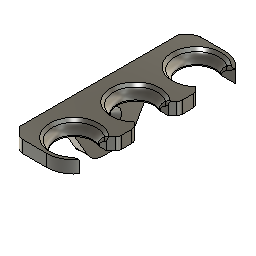
SKADIS_SNS_WeraMicro (Autodesk Fusion 360 design; units mm, degrees)
Autodesk Fusion 360 part; units mm, degrees
sketch "SlotLayout" plane through (0, 0, 0) normal (1, 0, 0) x (0, 1, 0)
  line L0 (-22.4, 25) -> (-22.4, 15)
  line L1 (82.4, 5) -> (82.4, -5)
  line L2 (-37.6, -5) -> (-37.6, 5)
  line L3 (-80, 5) -> (-80, -5) construction
  line L4 (-97.6, 15) -> (-97.6, 25)
  line L5 (2.4, -5) -> (2.4, 5)
  arc A0 (-77.6, 5) -> (-82.4, 5) centre (-80, 5) ccw
  arc A1 (22.4, 25) -> (17.6, 25) centre (20, 25) ccw
  arc A2 (-97.6, 25) -> (-102.4, 25) centre (-100, 25) ccw
  arc A3 (97.6, 15) -> (102.4, 15) centre (100, 15) ccw
  line L6 (-60, 25) -> (-60, 15) construction
  line L7 (-77.6, -5) -> (-77.6, 5)
  arc A4 (77.6, -5) -> (82.4, -5) centre (80, -5) ccw
  line L8 (-40, 5) -> (-40, -5) construction
  line L9 (-57.6, 15) -> (-57.6, 25)
  line L10 (-62.4, 25) -> (-62.4, 15)
  line L11 (-102.4, 25) -> (-102.4, 15)
  line L12 (97.6, 15) -> (97.6, 25)
  arc A5 (-102.4, 15) -> (-97.6, 15) centre (-100, 15) ccw
  line L13 (20, 25) -> (20, 15) construction
  line L14 (22.4, 25) -> (22.4, 15)
  line L15 (-80, 0) -> (0, 0) construction
  line L16 (62.4, 25) -> (62.4, 15)
  line L17 (42.4, 5) -> (42.4, -5)
  arc A6 (2.5, 5) -> (-2.5, 5) centre (0, 5) ccw
  arc A7 (2.4, 5) -> (-2.4, 5) centre (0, 5) ccw
  line L18 (80, 5) -> (80, -5) construction
  arc A8 (82.4, 5) -> (77.6, 5) centre (80, 5) ccw
  arc A9 (-2.5, -5) -> (2.5, -5) centre (0, -5) ccw
  arc A10 (57.6, 15) -> (62.4, 15) centre (60, 15) ccw
  arc A11 (62.4, 25) -> (57.6, 25) centre (60, 25) ccw
  line L19 (17.6, 15) -> (17.6, 25)
  line L20 (-20, 25) -> (-20, 15) construction
  line L21 (-42.4, 5) -> (-42.4, -5)
  line L22 (60, 25) -> (60, 15) construction
  arc A12 (42.4, 5) -> (37.6, 5) centre (40, 5) ccw
  line L23 (-100, 25) -> (-100, 15) construction
  line L24 (100, 25) -> (100, 15) construction
  arc A13 (-57.6, 25) -> (-62.4, 25) centre (-60, 25) ccw
  arc A14 (37.6, -5) -> (42.4, -5) centre (40, -5) ccw
  line L25 (40, 5) -> (40, -5) construction
  line L26 (-17.6, 15) -> (-17.6, 25)
  arc A15 (-17.6, 25) -> (-22.4, 25) centre (-20, 25) ccw
  line L27 (-82.4, 5) -> (-82.4, -5)
  line L28 (-2.5, 5) -> (-2.5, -5)
  line L29 (-2.4, 5) -> (-2.4, -5)
  line L30 (102.4, 25) -> (102.4, 15)
  arc A16 (17.6, 15) -> (22.4, 15) centre (20, 15) ccw
  arc A17 (-22.4, 15) -> (-17.6, 15) centre (-20, 15) ccw
  line L31 (37.6, -5) -> (37.6, 5)
  line L32 (0, 5) -> (0, -5) construction
  arc A18 (-62.4, 15) -> (-57.6, 15) centre (-60, 15) ccw
  arc A19 (-42.4, -5) -> (-37.6, -5) centre (-40, -5) ccw
  arc A20 (-2.4, -5) -> (2.4, -5) centre (0, -5) ccw
  arc A21 (102.4, 25) -> (97.6, 25) centre (100, 25) ccw
  arc A22 (-82.4, -5) -> (-77.6, -5) centre (-80, -5) ccw
  arc A23 (-37.6, 5) -> (-42.4, 5) centre (-40, 5) ccw
  line L33 (77.6, -5) -> (77.6, 5)
  line L34 (57.6, 15) -> (57.6, 25)
  line L35 (2.5, -5) -> (2.5, 5)
  point P0 (-20, 20)
  point P1 (-40, 0)
  dimension "d9" = -40
  dimension "d10" = 0
  dimension "d255" = 0.1
  dimension "d22" = 10
  dimension "d23" = 2.4
  dimension "d4" = 40
  dimension "d25" = 40
  dimension "d26" = 20
  dimension "d27" = 20
  constraint tangent L27 A22
  constraint tangent L7 A22
  constraint parallel L7 L27
  constraint tangent A0 L7
  constraint tangent A0 L27
  constraint vertical L3
  constraint tangent L21 A19
  constraint tangent L2 A19
  constraint parallel L2 L21
  constraint tangent L2 A23
  constraint tangent L21 A23
  constraint vertical L8
  constraint tangent L29 A20
  constraint tangent L5 A20
  constraint parallel L5 L29
  constraint tangent L5 A7
  constraint tangent A7 L29
  constraint parallel L2 L32
  constraint midpoint L15.start L3
  constraint midpoint L15.end L32
  constraint horizontal L15
  constraint equal L8 L32
  constraint equal L3 L8
  constraint midpoint P1 L8
  constraint coincident P1 L15
  constraint equal A7 A23
  constraint equal A0 A23
  constraint coincident L15.end origin
  constraint symmetric A0.end L1.start L32
  constraint symmetric L1.end L27.end L32
  constraint symmetric L7.start A4.start L32
  constraint symmetric A8.end A0.start L32
  constraint symmetric A4 L32 A22
  constraint symmetric A0 A8 L32
  constraint symmetric L17.start L21.start L32
  constraint symmetric L17.end L21.end L32
  constraint symmetric A14.start L2.start L32
  constraint symmetric A12.end L2.end L32
  constraint symmetric A14 L32 A19
  constraint symmetric A12 L32 A23
  constraint tangent L0 A17
  constraint tangent L26 A17
  constraint parallel L0 L26
  constraint tangent L26 A15
  constraint tangent L0 A15
  constraint vertical L20
  constraint equal L20 L32
  constraint equal A7 A15
  constraint midpoint P0 L20
  constraint symmetric L0.end L14.end L32
  constraint symmetric L26.end A1.end L32
  constraint symmetric L0.start A1.start L32
  constraint symmetric L26.start L19.start L32
  constraint symmetric A1 A15 L32
  constraint symmetric A16 A17 L32
  constraint symmetric A11.end L9.end L32
  constraint symmetric L16.start L10.start L32
  constraint symmetric A11 A13 L32
  constraint symmetric L16.end L10.end L32
  constraint symmetric A10.start L9.start L32
  constraint symmetric A10 L32 A18
  constraint symmetric L12.end L4.end L32
  constraint symmetric L30.start A2.end L32
  constraint symmetric A2 L32 A21
  constraint symmetric A3.end L11.end L32
  constraint symmetric A3.start L4.start L32
  constraint symmetric A3 A5 L32
  measures "d22" distance of A6.centre A9.centre
  measures "d23" radius of A7
  measures "d4" distance of L8 L32
  measures "d25" distance of L3 L8
  measures "d26" horizontal distance of L20.end A6.centre
  measures "d27" vertical distance of P0 L15.end
sketch "VerticalPrintKey" plane through (0, 0, 0) normal (1, 0, 0) x (0, 1, 0)
  line L0 (-2.6, 6.7) -> (2.6, 6.7)
  line L1 (2.6, 6.7) -> (2.6, -6.7)
  line L2 (2.6, -6.7) -> (-2.6, -6.7)
  line L3 (-2.6, -6.7) -> (-2.6, 6.7)
  line L4 (0, 6.7) -> (0, -6.7) construction
  circle A0 centre (0, 0) radius 1.6
  line L5 (2.6, 0) -> (20.8722, 0) construction
  line L6 (20.8722, 0) -> (11.7361, 9.1361) construction
  line L7 (11.7361, 9.1361) -> (11.7361, -9.1361) construction
  line L8 (11.7361, -9.1361) -> (20.8722, 0) construction
  dimension "d18" = 13.4
  dimension "d19" = 5.2
  dimension "d20" = 3.2
  constraint horizontal L0
  constraint vertical L1
  constraint horizontal L2
  constraint vertical L3
  constraint midpoint L0 L4.start
  constraint midpoint L2 L4.end
  constraint midpoint L4 A0.centre
  constraint coincident A0.centre origin
  constraint midpoint L1 L5.start
  constraint perpendicular L1 L5
  constraint perpendicular L5 L7
  constraint perpendicular L6 L8
  constraint midpoint L5 L7
  measures "d18" distance of L4.start L4.end
  measures "d19" distance of L1 L3
  measures "d20" diameter of A0
sketch "HorizontalPrintKey" plane through (0, 0, 0) normal (1, 0, 0) x (0, 1, 0)
  circle A0 centre (0, 0) radius 1.6
  line L0 (2.6, -6.7) -> (-2.6, -6.7)
  line L1 (-2.6, -6.7) -> (-2.6, 6.7)
  line L2 (-2.6, 6.7) -> (2.6, 6.7)
  line L3 (2.6, 6.7) -> (2.6, -6.7)
  line L4 (0, 6.7) -> (0, -6.7) construction
  line L5 (0, 6.7) -> (0, 23.5939) construction
  line L6 (0, 23.5939) -> (-8.4469, 15.1469) construction
  line L7 (-8.4469, 15.1469) -> (8.4469, 15.1469) construction
  line L8 (8.4469, 15.1469) -> (0, 23.5939) construction
  line L9 (17.4, -6.7) -> (17.4, 6.7)
  line L10 (17.4, 6.7) -> (22.6, 6.7)
  line L11 (22.6, -6.7) -> (17.4, -6.7)
  line L12 (22.6, 6.7) -> (22.6, -6.7)
  circle A1 centre (20, 0) radius 1.6
  line L13 (37.4, -6.7) -> (37.4, 6.7)
  line L14 (37.4, 6.7) -> (42.6, 6.7)
  line L15 (42.6, -6.7) -> (37.4, -6.7)
  line L16 (42.6, 6.7) -> (42.6, -6.7)
  circle A2 centre (40, 0) radius 1.6
  line L17 (-37.4, 6.7) -> (-42.6, 6.7)
  line L18 (-22.6, -6.7) -> (-17.4, -6.7)
  line L19 (-42.6, -6.7) -> (-37.4, -6.7)
  line L20 (-37.4, -6.7) -> (-37.4, 6.7)
  circle A3 centre (-40, 0) radius 1.6
  circle A4 centre (-20, 0) radius 1.6
  line L21 (-42.6, 6.7) -> (-42.6, -6.7)
  line L22 (-22.6, 6.7) -> (-22.6, -6.7)
  line L23 (-17.4, -6.7) -> (-17.4, 6.7)
  line L24 (-17.4, 6.7) -> (-22.6, 6.7)
  dimension "d21" = 13.4
  dimension "d24" = 5.2
  dimension "d28" = 3.2
  dimension "d32" = 20
  dimension "d33" = 0
  constraint horizontal L2
  constraint vertical L3
  constraint horizontal L0
  constraint vertical L1
  constraint midpoint L4.start L2
  constraint midpoint L4.end L0
  constraint midpoint A0.centre L4
  constraint coincident A0.centre origin
  constraint perpendicular L2 L5
  constraint perpendicular L5 L7
  constraint midpoint L5 L7
  constraint perpendicular L6 L8
  constraint symmetric L5 L9.start L18.end
  constraint symmetric L5 L9.end L23.end
  constraint symmetric L5 L10.end L22.start
  constraint symmetric L5 L11.start L18.start
  constraint symmetric L5 A1 A4
  constraint symmetric L5 L13.start L19.end
  constraint symmetric L5 L13.end L17.start
  constraint symmetric L5 L14.end L17.end
  constraint symmetric L5 L15.start L19.start
  constraint symmetric L5 A2 A3
  measures "d21" distance of L4.end L4.start
  measures "d24" distance of L1 L3
  measures "d28" diameter of A0
sketch "MainProfile " plane through (0, 0, 0) normal (0, 0, 1) x (1, 0, 0) in component "SNS_WeraMicro_x3"
  circle A0 centre (12, 20) radius 9 construction
  arc A1 (12, -29) -> (19.1239, -25.5) centre (12, -20) ccw
  line L0 (14.3979, -14.5) -> (19.1239, -14.5)
  line L1 (0, 29) -> (12, 29)
  line L2 (0, 0) -> (0, -29)
  line L3 (12, -20) -> (12, 20) construction
  circle A2 centre (12, -20) radius 9 construction
  line L4 (4, 29) -> (4, -29)
  line L5 (14.3979, 14.5) -> (19.1239, 14.5)
  line L6 (14.3979, 5.5) -> (19.1239, 5.5)
  arc A3 (19.1239, 25.5) -> (12, 29) centre (12, 20) ccw
  line L7 (14.3979, -25.5) -> (19.1239, -25.5)
  circle A4 centre (12, -20) radius 6
  line L8 (0, 0) -> (0, 29)
  line L9 (14.3979, -5.5) -> (19.1239, -5.5)
  line L10 (19.1239, -25.5) -> (19.1239, 25.5)
  line L11 (19.1239, 25.5) -> (14.3979, 25.5)
  line L12 (12, 0) -> (0, 0) construction
  circle A5 centre (12, 0) radius 9 construction
  line L13 (0, -29) -> (12, -29)
  circle A6 centre (12, 20) radius 6
  circle A7 centre (12, 0) radius 6
  dimension "d34" = 12
  dimension "d5" = 40
  dimension "d6" = 18
  dimension "d37" = 12
  dimension "d38" = 5.5
  dimension "d13" = 4
  constraint vertical L3
  constraint coincident L12.start L3
  constraint coincident L2.start L8.start
  constraint midpoint L12.start L3
  constraint horizontal L12
  constraint coincident A1.centre L3.start
  constraint coincident L12.start A5.centre
  constraint coincident A0.centre L3.end
  constraint equal A4 A7
  constraint equal A6 A7
  constraint concentric A2 A4
  constraint concentric A5 A7
  constraint concentric A0 A6
  constraint equal A0 A5
  constraint equal A2 A5
  constraint perpendicular L2 L12
  constraint coincident A1.start A2
  constraint tangent A2 L13
  constraint coincident L7.start A4
  constraint coincident A1.end A2
  constraint horizontal L7
  constraint coincident L0.start A4
  constraint coincident L0.end A2
  constraint horizontal L0
  constraint coincident L9.start A7
  constraint coincident L9.end A5
  constraint horizontal L9
  constraint coincident L6.start A7
  constraint coincident L6.end A5
  constraint parallel L6 L9
  constraint coincident A3.start A0
  constraint perpendicular L7 L10
  constraint coincident L6.end L10
  constraint coincident L9.end L10
  constraint coincident L0.end L10
  constraint coincident L5.start A6
  constraint coincident L5.end L10
  constraint perpendicular L5 L10
  constraint coincident L5.end A0
  constraint perpendicular L10 L11
  constraint horizontal L13
  constraint tangent A1 L13
  constraint perpendicular L8 L12
  constraint coincident L1.end A0
  constraint horizontal L1
  constraint tangent A0 L1
  constraint tangent L1 A3
  constraint coincident L4.start L1
  constraint coincident L4.end L13
  constraint perpendicular L4 L13
  constraint coincident L11.end A6
  measures "d34" diameter of A4
  measures "d5" distance of A1.centre A0.centre
  measures "d6" diameter of A2
  measures "d37" distance of L2.start L12.start
  measures "d38" distance of A1.centre L7
  measures "d13" distance of L2 L4
extrude "Extrude1" add sketch "MainProfile " along normal mid plane 18 contours L1 L2 L4 L8 L13 in component "SNS_WeraMicro_x3"
extrude "Extrude2" add sketch "MainProfile " against normal blind 4 from surface at 9 contours A1 L0 L1 L4 L5 L6 A3 L7 A4 L9 L10 L11 L13 A6 A7 in component "SNS_WeraMicro_x3"
chamfer "Chamfer1" distance 2 angle 45 3 edges at (6, 20, 9) (6, 0, 9) (6, -20, 9) in component "SNS_WeraMicro_x3"
fillet "Fillet1" radius 4 3 edges at (6, -20, 7) (6, 0, 7) (6, 20, 7) in component "SNS_WeraMicro_x3"
fillet "Fillet2" radius 1.2 18 edges at (14.3979, -14.5, 5.1716) (15.1765, -14.5, 6.9811) (17.1799, -14.5, 8.5552) (17.1799, -25.5, 8.5552) (15.1765, -25.5, 6.9811) (14.3979, -25.5, 5.1716) (14.3979, 5.5, 5.1716) (15.1765, 5.5, 6.9811) (17.1799, 5.5, 8.5552) (17.1799, -5.5, 8.5552) (15.1765, -5.5, 6.9811) (14.3979, -5.5, 5.1716) (17.1799, 14.5, 8.5552) (15.1765, 14.5, 6.9811) (14.3979, 14.5, 5.1716) (14.3979, 25.5, 5.1716) (15.1765, 25.5, 6.9811) (17.1799, 25.5, 8.5552) in component "SNS_WeraMicro_x3"
extrude "Extrude3" cut sketch "HorizontalPrintKey" along normal blind 1.2 contours A0 | L0 L1 L2 L3 in component "SNS_WeraMicro_x3"
extrude "Extrude4" cut sketch "HorizontalPrintKey" along normal blind 18 contours A0 in component "SNS_WeraMicro_x3"
chamfer "Chamfer3" distance 1.8 distance2 1.8 1 edges at (4, -1.4917, 0.5786) measured on face at (4, -19.8607, -1.4128) in component "SNS_WeraMicro_x3"
sketch "Sketch3" plane through (4, 0, 0) normal (1, 0, 0) x (0, 1, 0) in component "SNS_WeraMicro_x3"
  line L0 (29, 5) -> (-29, 5)
  line L1 (-29, 5) -> (-29, -9)
  line L2 (-29, -9) -> (29, -9)
  line L3 (29, -9) -> (29, 5)
  circle A0 centre (0, 0) radius 3.4
  line L4 (0, -9) -> (0, 5) construction
  line L5 (-6, -9) -> (-6, 5)
  line L6 (6, -9) -> (6, 5)
  line L7 (-6, -9) -> (-14.0829, 5)
  line L8 (6, -9) -> (14.0829, 5)
  dimension "d73" = 6
  dimension "d85" = 30
  dimension "d86" = 30
  constraint midpoint L2 L4.start
  constraint midpoint L0 L4.end
  constraint coincident L0 L5.end
  constraint perpendicular L0 L5
  constraint symmetric L4 L5.start L6.start
  constraint symmetric L4 L5.end L6.end
  constraint coincident L2 L6.start
  constraint coincident L0 L7.end
  constraint coincident L0 L8.end
  measures "d73" distance of L4 L5.start
  measures "d85" angle of L5 L7
  measures "d86" angle of L6 L8
extrude "Extrude5" cut sketch "Sketch3" against normal through all contours L0 L2 L3 L8 | L0 L1 L2 L7 in component "SNS_WeraMicro_x3"
chamfer "Chamfer7" distance 3 distance2 3 2 edges at (0, -29, 7) (0, 29, 7) measured on face at (0, -6.4276, 1.6667) measured on face at (4, 29, 7.6667) in component "SNS_WeraMicro_x3"
chamfer "Chamfer7" distance 2 distance2 2 4 edges at (19.1239, -14.5, 7) (19.1239, -5.5, 7) (19.1239, 5.5, 7) (19.1239, 14.5, 7) measured on face at (19.1239, -11.5, 7.6667) measured on face at (18.3609, -5.5, 7.2107) measured on face at (19.1239, 8.5, 6.3333) measured on face at (18.3609, 14.5, 7.2107) in component "SNS_WeraMicro_x3"
chamfer "Chamfer7" distance 1.5 angle 45 1 edges at (4, 0, 5) in component "SNS_WeraMicro_x3"
fillet "Fillet6" radius 6 2 edges at (2, -6, -9) (2, 6, -9) in component "SNS_WeraMicro_x3"
fillet "Fillet6" radius 3 2 edges at (3, -29, 7) (3, 29, 7) in component "SNS_WeraMicro_x3"
fillet "Fillet6" radius 2 4 edges at (19.1239, -12.5, 7) (19.1239, -7.5, 7) (19.1239, 12.5, 7) (19.1239, 7.5, 7) in component "SNS_WeraMicro_x3"
component "SNS_WeraMicro_x3" placed x (1, 0, 0) y (0, 1, 0) z (0, 0, 1) at (0, 0, 0)
equation "XY_Tolerance = 0.2 mm"
equation "Z_Tolerance = 0.2 mm"
equation "Wall_Thickness = 0.4 mm"
equation "Layer_Height = 0.2 mm"
equation "M3Hole_wClearance = 3.2 mm"
equation "M3Hole_wSelfTapping = 2.8 mm"
equation "d20 = M3Hole_wClearance"
equation "d28 = M3Hole_wClearance"
equation "M3Hole_CounterSink = 1.8 mm"
equation "d56 = M3Hole_CounterSink"
named bodies: "WeraMicro_x3"
